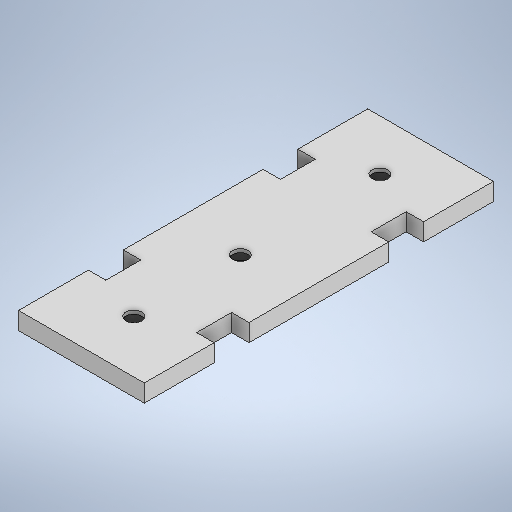
# Autodesk Inventor part: Part1v3
Saved by Autodesk Inventor 2025.2 (Build 292293000, 293)
## iProperties
Created: 2025-03-26
Part Number: Part1v3
Material: Generic
Document SubType Name: Sheet Metal
Designer: ziyuz
Density: 1 g/cm^3
Sheet Metal Rule: Default_mm
Appearance: Default
Author: ziyuz
Autodesk Inventor part; units mm, degrees
ref_plane "YZ Plane" through (0, 0, 0) normal (1, 0, 0) x (0, 1, 0)
ref_plane "XZ Plane" through (0, 0, 0) normal (0, 1, 0) x (-1, 0, 0)
ref_plane "XY Plane" through (0, 0, 0) normal (0, 0, 1) x (1, 0, 0)
sketch "Sketch2" plane through (0, 0, 0) normal (0, 1, 0) x (-1, 0, 0)
  line L0 (0, 0) -> (-36, 0)
  line L1 (-36, 0) -> (-36, -100)
  line L2 (-36, -100) -> (0, -100)
  line L3 (0, -100) -> (0, 0)
  line L4 (-36, 0) -> (-36, -20)
  line L5 (-36, -20) -> (0, -20)
  line L6 (-36, -100) -> (-36, -80)
  line L7 (-36, -80) -> (-36, -61.7109)
  line L8 (0, -61.7109) -> (0, -80)
  line L9 (-36, -80) -> (-36, -70)
  line L10 (-36, -70) -> (0, -70)
  line L11 (0, -80) -> (-36, -80)
  line L12 (0, -70) -> (0, -80)
  line L13 (0, -70) -> (-5, -70)
  line L14 (-5, -70) -> (-5, -80)
  line L15 (-36, -20) -> (-36, -30)
  line L16 (-36, -30) -> (0, -30)
  line L17 (0, -20) -> (-5, -20)
  line L18 (-5, -20) -> (-5, -30)
  line L19 (-36, -80) -> (-31, -80)
  line L20 (-31, -80) -> (-31, -70)
  line L21 (-31, -30) -> (-31, -20)
  line L22 (-18, 0) -> (-18, -15)
  line L23 (-18, -15) -> (-18, -45.5)
  circle A0 centre (-18, -45.5) radius 5.05
  line L24 (-18, -45.5) -> (-18, -85.5)
  circle A1 centre (-18, -85.5) radius 5.05
  circle A2 centre (-18, -15) radius 5
  dimension "d0" = 36
  dimension "d1" = 100
  dimension "d2" = 20
  dimension "d3" = 20
  dimension "d4" = 10
  dimension "d5" = 5
  dimension "d6" = 10
  dimension "d7" = 5
  dimension "d8" = 5
  dimension "d9" = 15
  dimension "d11" = 30.5
  dimension "d12" = 10.1
  dimension "d13" = 40
  dimension "d14" = 10.1
  constraints: 50 end point, 19 point on line, 8 perpendicular, 4 coincident, 3 centre point, 3 parallel, 3 vertical, 1 horizontal, 1 midpoint
  measures "d0" distance of L2.end L1.end
  measures "d1" distance of L1.end L0.end
  measures "d2" distance of L0.end L4.end
  measures "d3" distance of L1.end L6.end
  measures "d4" distance of L6.end L9.end
  measures "d5" distance of L10.end L13.end
  measures "d6" distance of L4.end L15.end
  measures "d7" distance of L5.end L17.end
  measures "d8" distance of L6.end L19.end
  measures "d9" distance of L22.start L22.end
  measures "d11" distance of L23.start L23.end
  measures "d12" diameter of A0
  measures "d13" distance of L24.start L24.end
  measures "d14" diameter of A1
extrude "Extrusion1" add sketch "Sketch2" along normal blind 5 contours L3 L5 A2 L22 L0 | L22 A2 L5 L1 L0 | L3 L10 L24 A0 L23 L16 | L18 L16 L23 L5 | L23 L16 L21 L5 | L16 L23 A0 L24 L10 L1 | L3 L2 L1 L11 | L14 L11 L24 L10 | L24 L11 L20 L10
sketch "Sketch3" plane through (0, 5, 0) normal (0, 1, 0) x (1, 0, 0)
  circle A0 centre (18, 15) radius 5 projected
  circle A1 centre (18, 15) radius 5
  circle A2 centre (18, 45.5) radius 5.05 projected
  circle A3 centre (18, 45.5) radius 5.05
  circle A4 centre (18, 85.5) radius 5.05 projected
  circle A5 centre (18, 85.5) radius 5.05
  circle A6 centre (18, 45.5) radius 2.25
  circle A7 centre (18, 85.5) radius 2.25
  circle A8 centre (18, 15) radius 2.25
  point P0 (0, 0)
  dimension "d18" = 4.5
  dimension "d19" = 4.5
  dimension "d20" = 4.5
  constraints: 6 centre point, 6 coincident
  measures "d18" diameter of A6
  measures "d19" diameter of A7
  measures "d20" diameter of A8
extrude "Extrusion2" add sketch "Sketch3" against normal blind 1
equation "\"BendRadius\" = Thickness"
equation "\"BendReliefWidth\" = Thickness"
equation "\"BendReliefDepth\" = 0.5 * Thickness"
equation "\"CornerReliefSize\" = 4 * Thickness"
equation "\"MinimumRemnant\" = 2 * Thickness"
equation "\"TransitionRadius\" = BendRadius"
equation "\"JacobiRadiusSize\" = BendRadius"
equation "\"GapSize\" = Thickness"
equation "\"Thickness\" = 0.5"
body "Solid1"
